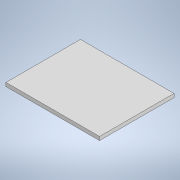
# Autodesk Inventor part: BottomPlate
Saved by Autodesk Inventor 2022.2 (Build 262287010, 287A)
## iProperties
Created: 2022-07-12
Part Number: BottomPlate
Material: Generic
Document SubType Name: Modeling
Designer: keaton
Density: 1 g/cm^3
Appearance: Default
Author: keaton
Autodesk Inventor part; units mm, degrees
ref_plane "YZ Plane" through (0, 0, 0) normal (1, 0, 0) x (0, 1, 0)
ref_plane "XZ Plane" through (0, 0, 0) normal (0, 1, 0) x (-1, 0, 0)
ref_plane "XY Plane" through (0, 0, 0) normal (0, 0, 1) x (1, 0, 0)
sketch "DeckFace" plane through (0, 0, 0) normal (0, 1, 0) x (-1, 0, 0)
  line L0 (-47.5, 37) -> (47.5, 37)
  line L1 (47.5, 37) -> (47.5, -37)
  line L2 (47.5, -37) -> (-47.5, -37)
  line L3 (-47.5, -37) -> (-47.5, 37)
  line L4 (-47.5, 37) -> (47.5, -37) construction
  line L5 (47.5, 37) -> (-47.5, -37) construction
  line L6 (51.5, -41) -> (51.5, 41)
  line L7 (51.5, 41) -> (-51.5, 41)
  line L8 (-51.5, 41) -> (-51.5, -41)
  line L9 (-51.5, -41) -> (51.5, -41)
  point P0 (0, 0)
  dimension "d4" = 4
  measures "d4" distance between parallel lines of L1 L6
extrude "Stock" add sketch "DeckFace" along normal blind 4 contours L0 L1 L2 L3 | L9 L8 L7 L6
equation "\"d4\" = PlateThickness"
equation "\"d5\" = PlateThickness"
equation "\"PlateThickness\" = 4"
body "Solid1"
